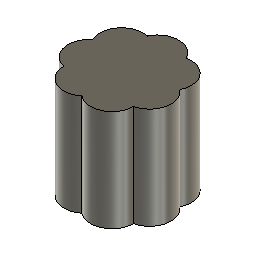
knob (Autodesk Fusion 360 design; units mm, degrees)
Autodesk Fusion 360 part; units mm, degrees
sketch "Sketch2" plane through (0, 0, 0) normal (0, 0, 1) x (1, 0, 0)
  circle A0 centre (0, 0) radius 8.5
  circle A1 centre (0, 0) radius 3
  circle A2 centre (0, 5) radius 3.5
  circle A3 centre (-3.9092, 3.1174) radius 3.5
  circle A4 centre (-4.8746, -1.1126) radius 3.5
  circle A5 centre (-2.1694, -4.5048) radius 3.5
  circle A6 centre (2.1694, -4.5048) radius 3.5
  circle A7 centre (4.8746, -1.1126) radius 3.5
  circle A8 centre (3.9092, 3.1174) radius 3.5
  circle A9 centre (-3.9092, 3.1174) radius 3.5
  circle A10 centre (-2.1694, -4.5048) radius 3.5
  circle A11 centre (4.8746, -1.1126) radius 3.5
  circle A12 centre (-4.8746, -1.1126) radius 3.5
  circle A13 centre (0, 5) radius 3.5
  circle A14 centre (0, 0) radius 8.5
  circle A15 centre (0, 0) radius 3
  circle A16 centre (2.1694, -4.5048) radius 3.5
  circle A17 centre (2.1694, -4.5048) radius 2.5
  circle A18 centre (4.8746, -1.1126) radius 2.5
  circle A19 centre (3.9092, 3.1174) radius 2.5
  circle A20 centre (0, 5) radius 2.5
  circle A21 centre (-3.9092, 3.1174) radius 2.5
  circle A22 centre (-4.8746, -1.1126) radius 2.5
  circle A23 centre (-2.1694, -4.5048) radius 2.5
  point P0 (3.9092, 3.1174)
  dimension "d3" = 17
  dimension "d5" = 6
  dimension "d6" = 7
  dimension "d16" = 17
  dimension "d17" = 6
  dimension "d18" = 7
  dimension "d19" = 5
  dimension "d20" = 5
  dimension "d21" = 5
  dimension "d22" = 5
  dimension "d23" = 5
  dimension "d24" = 5
  dimension "d25" = 5
  constraint coincident A0.centre A1.centre
  constraint concentric A0 A1
  constraint concentric A14 A15
  constraint concentric A6 A17
  constraint concentric A7 A18
  constraint concentric A8 A19
  constraint concentric A2 A20
  constraint concentric A3 A21
  constraint concentric A12 A22
  constraint concentric A10 A23
  measures "d3" diameter of A0
  measures "d5" diameter of A1
  measures "d6" diameter of A2
  measures "d16" diameter of A14
  measures "d17" diameter of A15
  measures "d18" diameter of A13
  measures "d19" diameter of A17
  measures "d20" diameter of A18
  measures "d21" diameter of A19
  measures "d22" diameter of A20
  measures "d23" diameter of A21
  measures "d24" diameter of A22
  measures "d25" diameter of A23
extrude "Extrude1" add sketch "Sketch2" along normal blind 9 contours A2 A7 A8 A11 A13 A19 | A0 A6 A7 A8 A11 A14 A16 A18 | A2 A3 A8 A9 A13 A20 | A2 A8 A13 A19 A20 | A2 A3 A4 A9 A12 A13 A21 | A2 A3 A9 A13 A20 A21 | A7 A8 A11 A18 A19 | A1 A2 A7 A11 A13 A15 A19 | A1 A2 A13 A15 A19 A20 | A1 A8 A15 A19 A20 | A1 A3 A8 A9 A15 A20 | A5 A6 A7 A10 A11 A16 A17 | A6 A7 A11 A16 A17 A18 | A0 A3 A4 A5 A9 A10 A12 A14 A22 | A3 A4 A9 A12 A21 A22 | A1 A2 A13 A15 A20 A21 | A1 A2 A4 A12 A13 A15 A21 | A1 A3 A9 A15 A20 A21 | A1 A7 A11 A15 A18 A19 | A1 A6 A8 A15 A16 A18 | A1 A8 A15 A18 A19 | A19 A20 | A1 A3 A8 A9 A15 A20 | A1 A8 A15 A20 | A4 A5 A6 A10 A12 A16 A23 | A5 A6 A10 A16 A17 A23 | A1 A5 A7 A10 A11 A15 A17 | A1 A7 A11 A15 A17 A18 | A1 A3 A9 A15 A21 A22 | A1 A3 A5 A9 A10 A15 A22 | A1 A4 A12 A15 A21 A22 | A1 A2 A4 A12 A13 A15 A21 | A1 A2 A13 A15 A21 | A20 A21 | A1 A2 A7 A11 A13 A15 A19 | A1 A7 A11 A15 A19 | A18 A19 | A1 A8 A15 A18 | A1 A6 A8 A15 A16 A18 | A1 A2 A13 A15 A19 | A1 A15 A19 A20 | A1 A2 A8 A13 A15 A19 A20 | A1 A3 A9 A15 A20 | A2 A3 A8 A9 A13 A20 | A4 A5 A10 A12 A22 A23 | A1 A5 A10 A15 A17 A23 | A1 A4 A6 A12 A15 A16 A23 | A1 A6 A15 A16 A17 A23 | A1 A6 A15 A16 A17 A18 | A1 A7 A11 A15 A17 | A1 A5 A7 A10 A11 A15 A17 | A1 A3 A5 A9 A10 A15 A22 | A1 A3 A9 A15 A22 | A21 A22 | A1 A5 A10 A15 A22 A23 | A1 A4 A12 A15 A21 | A1 A15 A20 A21 | A1 A2 A3 A9 A13 A15 A20 A21 | A2 A3 A4 A9 A12 A13 A21 | A1 A15 A18 A19 | A1 A7 A8 A11 A15 A18 A19 | A2 A7 A8 A11 A13 A19 | A1 A6 A15 A16 A18 | A6 A7 A8 A11 A16 A18 | A2 A3 A4 A5 A6 A7 A8 A9 A10 A11 A12 A13 A16 | A1 A4 A12 A15 A22 A23 | A17 A23 | A1 A6 A15 A16 A23 | A1 A4 A6 A12 A15 A16 A23 | A17 A18 | A1 A5 A10 A15 A17 | A1 A6 A7 A11 A15 A16 A17 A18 | A1 A15 A17 A18 | A5 A6 A7 A10 A11 A16 A17 | A1 A15 A21 A22 | A1 A3 A4 A9 A12 A15 A21 A22 | A1 A5 A10 A15 A22 | A3 A4 A5 A9 A10 A12 A22 | A22 A23 | A1 A4 A12 A15 A23 | A1 A15 A17 A23 | A1 A5 A6 A10 A15 A16 A17 A23 | A4 A5 A6 A10 A12 A16 A23 | A1 A4 A5 A10 A12 A15 A22 A23 | A1 A15 A22 A23 picked at (6.9816, 2.381) picked at (7.3287, 0.8776) picked at (0.2224, 8.1531) picked at (2.7619, 5.9299) picked at (-6.2357, 5.2573) picked at (-2.9142, 5.8566) picked at (6.3958, 1.3731) picked at (4.6445, 3.7483) picked at (1.9285, 2.707) picked at (0.915, 3.2085) picked at (-0.0712, 6) picked at (3.3371, -7.4422) picked at (5.1638, -3.9861) picked at (-7.899, -2.0317) picked at (-6.3958, 1.3731) picked at (-1.938, 2.7159) picked at (-4.6423, 3.7789) picked at (-0.9254, 3.3014) picked at (3.079, 1.2851) picked at (5.8237, -1.3854) picked at (3.3335, 0.1519) picked at (1.8711, 4.1299) picked at (0.2373, 2.7764) picked at (0.5959, 2.7362) picked at (-3.7379, -7.2492) picked at (0.0845, -6.541) picked at (2.5312, -5.471) picked at (2.2165, -2.4937) picked at (-3.3317, 0.1781) picked at (-5.8489, -1.2734) picked at (-3.079, 1.2851) picked at (-2.3187, 1.5455) picked at (-1.7677, 2.1719) picked at (-2.038, 3.9875) picked at (2.3187, 1.5455) picked at (2.5108, 1.2401) picked at (4.0717, 1.0212) picked at (2.8002, -0.0253) picked at (2.7596, -0.3864) picked at (1.7677, 2.1719) picked at (1.3427, 2.7458) picked at (1.0228, 2.3187) picked at (-0.5959, 2.7362) picked at (-0.051, 1.8412) picked at (-5.1667, -4.0122) picked at (0.4774, -5.7524) picked at (-2.6511, -5.3668) picked at (-0.5677, -3.2878) picked at (2.9244, -1.6061) picked at (1.7241, -2.2067) picked at (1.4185, -2.3985) picked at (-2.654, -0.8492) picked at (-2.8002, -0.0279) picked at (-4.0717, 1.0212) picked at (-2.9244, -1.6061) picked at (-2.5108, 1.2401) picked at (-1.3096, 2.7618) picked at (-1.1751, 2.2453) picked at (-1.4713, 1.1081) picked at (2.9758, 0.6981) picked at (2.4505, 0.646) picked at (1.4077, 1.1878) picked at (2.535, -1.1898) picked at (1.7836, -0.4594) picked at (-0.5275, -0.1824) picked at (-2.2165, -2.4937) picked at (-0.1056, -4.5048) picked at (-0.6503, -2.7238) picked at (-1.4185, -2.3985) picked at (3.3371, -2.5467) picked at (0.6503, -2.7238) picked at (1.9276, -1.6453) picked at (2.4011, -1.8913) picked at (0.8448, -1.6367) picked at (-2.9758, 0.6981) picked at (-2.4505, 0.646) picked at (-2.5366, -1.2123) picked at (-1.8063, -0.36) picked at (-3.7069, -3.0708) picked at (-1.7241, -2.2067) picked at (0.0184, -3.0565) picked at (-0.0845, -2.5328) picked at (-0.8448, -1.6367) picked at (-2.0347, -1.5243) picked at (-2.4011, -1.8913)
extrude "Extrude2" add 1 faces at (-1.5155, 1.2086, 9) along direction (0, 0, 1) blind 6
hole "Hole1" at (0.0633, 0.1229, 15) direction (0, 0, -1) diameter 6.1 depth 11 tip angle 180
move_body "Move1" bodies 1 to x (-1, 0, 0) y (0, 1, 0) z (0, 0, -1) at (0.1266, 0, 30)
move_body "Move2" bodies 1 to x (1, 0, 0) y (0, 1, 0) z (0, 0, 1) at (0, 0, -15)
extrude "Extrude3" cut sketch "Sketch2" along normal blind 2.75 contours A1 A2 A7 A11 A13 A15 A19 | A1 A2 A13 A15 A19 A20 | A1 A8 A15 A19 A20 | A1 A3 A8 A9 A15 A20 | A1 A2 A13 A15 A20 A21 | A1 A2 A4 A12 A13 A15 A21 | A1 A3 A9 A15 A20 A21 | A1 A7 A11 A15 A18 A19 | A1 A6 A8 A15 A16 A18 | A1 A8 A15 A18 A19 | A19 A20 | A1 A5 A7 A10 A11 A15 A17 | A1 A7 A11 A15 A17 A18 | A1 A3 A9 A15 A21 A22 | A1 A3 A5 A9 A10 A15 A22 | A1 A4 A12 A15 A21 A22 | A20 A21 | A18 A19 | A1 A15 A19 A20 | A1 A5 A10 A15 A17 A23 | A1 A4 A6 A12 A15 A16 A23 | A1 A6 A15 A16 A17 A23 | A1 A6 A15 A16 A17 A18 | A21 A22 | A1 A5 A10 A15 A22 A23 | A1 A15 A20 A21 | A1 A15 A18 A19 | A1 A4 A12 A15 A22 A23 | A17 A23 | A17 A18 | A1 A15 A17 A18 | A1 A15 A21 A22 | A22 A23 | A1 A15 A17 A23 | A1 A15 A22 A23 picked at (4.6445, 3.7483) picked at (1.9285, 2.707) picked at (0.915, 3.2085) picked at (-0.0712, 6) picked at (-1.938, 2.7159) picked at (-4.6423, 3.7789) picked at (-0.9254, 3.3014) picked at (3.079, 1.2851) picked at (5.8237, -1.3854) picked at (3.3335, 0.1519) picked at (1.8711, 4.1299) picked at (2.5312, -5.471) picked at (2.2165, -2.4937) picked at (-3.3317, 0.1781) picked at (-5.8489, -1.2734) picked at (-3.079, 1.2851) picked at (-2.038, 3.9875) picked at (4.0717, 1.0212) picked at (1.3427, 2.7458) picked at (0.4774, -5.7524) picked at (-2.6511, -5.3668) picked at (-0.5677, -3.2878) picked at (2.9244, -1.6061) picked at (-4.0717, 1.0212) picked at (-2.9244, -1.6061) picked at (-1.3096, 2.7618) picked at (2.9758, 0.6981) picked at (-2.2165, -2.4937) picked at (-0.1056, -4.5048) picked at (3.3371, -2.5467) picked at (2.4011, -1.8913) picked at (-2.9758, 0.6981) picked at (-3.7069, -3.0708) picked at (0.0184, -3.0565) picked at (-2.4011, -1.8913)
extrude "Extrude4" cut 1 faces at (-0.9222, -0.8364, 15) along direction (0, 0, -1) blind 1
extrude "Extrude5" add 1 faces at (6.5147, 1.4773, 0) along direction (0, 0, -1) blind 2
extrude "Extrude6" cut 1 faces at (-0.9222, -0.8364, 14) along direction (0, 0, -1) blind 1.5
extrude "Extrude7" add 1 faces at (6.5147, 1.4773, -2) along direction (0, 0, -1) blind 1
extrude "Extrude8" add 1 faces at (6.5147, 1.4773, -3) along direction (0, 0, -1) blind 1
